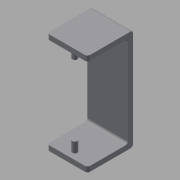
# Autodesk Inventor part: Bracket3
Saved by Autodesk Inventor 2017 (Build 210142000, 142)
## iProperties
Created: 2017-05-07
Part Number: Bracket3
Material: Generic
Document SubType Name: Modeling
Designer: zallen
Density: 1 g/cm^3
Appearance: Default
Author: zallen
Autodesk Inventor part; units mm, degrees
ref_plane "YZ Plane" through (0, 0, 0) normal (1, 0, 0) x (0, 1, 0)
ref_plane "XZ Plane" through (0, 0, 0) normal (0, 1, 0) x (-1, 0, 0)
ref_plane "XY Plane" through (0, 0, 0) normal (0, 0, 1) x (1, 0, 0)
sketch "Sketch1" plane through (0, 0, 0) normal (0, 0, 1) x (1, 0, 0)
  line L0 (25.4, -63.5) -> (-25.4, -63.5)
  line L1 (-25.4, -63.5) -> (-25.4, 63.5)
  line L2 (-25.4, 63.5) -> (25.4, 63.5)
  line L3 (25.4, 63.5) -> (25.4, -63.5)
  point P0 (0, 0)
  dimension "d0" = 50.8
  dimension "d1" = 127
  dimension "d2" = 63.5
  dimension "d3" = 25.4
  constraints: 8 end point, 2 parallel, 1 horizontal, 1 perpendicular
  measures "d0" distance of L0.start L0.end
  measures "d1" distance of L2.end L0.start
  measures "d2" distance from line of L0 point (0, 0)
  measures "d3" distance from line of L3 point (0, 0)
extrude "Extrusion1" add sketch "Sketch1" along normal blind 6.35
sketch "Sketch2" plane through (0, 0, 6.35) normal (0, 0, 1) x (1, 0, 0)
  line L0 (25.4, -63.5) -> (25.4, 63.5) projected
  line L1 (25.4, 63.5) -> (-25.4, 63.5)
  line L2 (-25.4, 63.5) -> (-25.4, 57.15)
  line L3 (-25.4, 57.15) -> (25.4, 57.15)
  line L4 (25.4, 57.15) -> (25.4, 63.5)
  line L5 (25.4, -63.5) -> (-25.4, -63.5)
  line L6 (-25.4, -63.5) -> (-25.4, -57.15)
  line L7 (-25.4, -57.15) -> (25.4, -57.15)
  line L8 (25.4, -57.15) -> (25.4, -63.5)
  point P0 (0, 0)
  dimension "d6" = 50.8
  dimension "d7" = 6.35
  dimension "d8" = 50.8
  dimension "d9" = 6.35
  constraints: 16 end point, 4 parallel, 2 horizontal, 2 perpendicular, 1 point on line
  measures "d6" distance of L3.end L2.end
  measures "d7" distance of L2.end L1.end
  measures "d8" distance of L6.end L7.end
  measures "d9" distance of L5.end L6.end
extrude "Extrusion2" add sketch "Sketch2" along normal blind 50.8
fillet "Fillet1" radius 3.175 8 edges at (-25.4, 60.325, 57.15) (25.4, 60.325, 57.15) (-25.4, -60.325, 57.15) (25.4, -60.325, 57.15) (0, -63.5, 0) (0, 63.5, 0) (0, 57.15, 6.35) (0, -57.15, 6.35)
sketch "Sketch3" plane through (-25.4, 57.15, 9.525) normal (0, -1, 0) x (1, 0, 0)
  circle A0 centre (25.4, 38.0964) radius 3.175
  line L0 (0, -6.35) -> (0, 44.45) projected
  line L1 (0, -0.0036) -> (75.5058, -0.0036) construction
  point P0 (25.4, -9.525)
  dimension "d13" = 6.35
  dimension "d14" = 25.4
  dimension "d15" = 38.1
  constraints: 2 end point, 1 centre point, 1 horizontal, 1 point on line
  measures "d13" diameter of A0
  measures "d14" distance from line of L0 A0.centre
  measures "d15" distance from line of L1 A0.centre
extrude "Extrusion3" add sketch "Sketch3" along normal blind 12.7
sketch "Sketch4" plane through (-25.4, -57.15, 9.525) normal (0, 1, 0) x (1, 0, 0)
  circle A0 centre (25.4, -38.1) radius 3.175
  line L0 (0, 0) -> (100.0722, 0) construction
  line L1 (0, 6.35) -> (0, -44.45) construction
  point P0 (25.4, 9.525)
  dimension "d18" = 6.35
  dimension "d19" = 38.1
  dimension "d20" = 25.4
  constraints: 2 end point, 1 centre point, 1 horizontal
  measures "d18" diameter of A0
  measures "d19" distance from line of L0 A0.centre
  measures "d20" distance from line of L1 A0.centre
extrude "Extrusion4" add sketch "Sketch4" along normal blind 12.7
body "Solid1"
